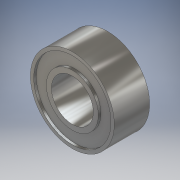
# Autodesk Inventor part: Ball Bearing 5 x 10 x 4.2
Saved by Autodesk Inventor 2019 (Build 230136000, 136)
## iProperties
Created: 2020-11-22
Part Number: Ball Bearing 5 x 10 x 4.2
Material: Stainless Steel
Document SubType Name: Modeling
Designer: asus
Density: 8 g/cm^3
Appearance: Chrome - Polished
Author: asus
Autodesk Inventor part; units mm, degrees
ref_plane "YZ Plane" through (0, 0, 0) normal (1, 0, 0) x (0, 1, 0)
ref_plane "XZ Plane" through (0, 0, 0) normal (0, 1, 0) x (-1, 0, 0)
ref_plane "XY Plane" through (0, 0, 0) normal (0, 0, 1) x (1, 0, 0)
sketch "Sketch1" plane through (0, 0, 0) normal (1, 0, 0) x (0, 1, 0)
  line L0 (4, 0) -> (2.5, 0)
  line L1 (2.5, 0) -> (3.1, 0)
  line L2 (3.1, 0) -> (3.1, -0.3)
  line L3 (3.1, -0.3) -> (4.6, -0.3)
  line L4 (4.6, -0.3) -> (4.6, 0)
  line L5 (4.6, 0) -> (5, 0)
  line L6 (5, 0) -> (5, -4.2)
  line L7 (5, -4.2) -> (4.6, -4.2)
  line L8 (4.6, -4.2) -> (4.6, -3.9)
  line L9 (4.6, -3.9) -> (3.1, -3.9)
  line L10 (3.1, -3.9) -> (3.1, -4.2)
  line L11 (3.1, -4.2) -> (2.5, -4.2)
  line L12 (2.5, -4.2) -> (2.5, 0)
  line L13 (0, 0) -> (0, -4.97)
  constraints: 28 end point, 1 vertical
revolve "Revolution1" add sketch "Sketch1" angle 360 about axis through (0, 0, 0) along (0, 0, -1)
body "Solid1"
